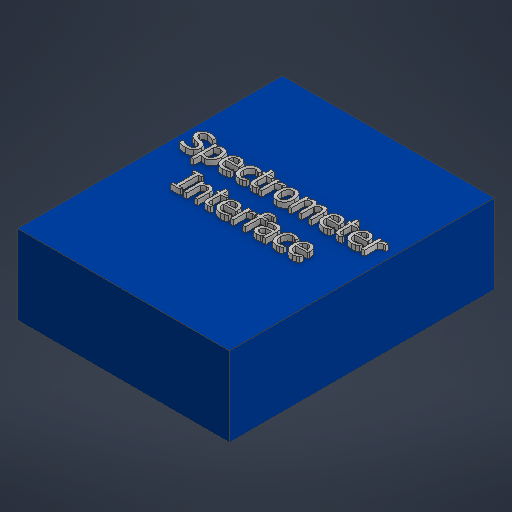
# Autodesk Inventor part: SpectrometerMeasurer
Saved by Autodesk Inventor 2025.1 (Build 291241000, 241)
## iProperties
Created: 2024-10-04
Part Number: SpectrometerMeasurer
Material: Generic
Document SubType Name: Modeling
Designer: jerem
Density: 1 g/cm^3
Appearance: Default
Author: jerem
Autodesk Inventor part; units mm, degrees
ref_plane "YZ Plane" through (0, 0, 0) normal (1, 0, 0) x (0, 1, 0)
ref_plane "XZ Plane" through (0, 0, 0) normal (0, 1, 0) x (-1, 0, 0)
ref_plane "XY Plane" through (0, 0, 0) normal (0, 0, 1) x (1, 0, 0)
sketch "Sketch1" plane through (0, 0, 0) normal (0, 1, 0) x (-1, 0, 0)
  line L0 (-40, -50) -> (40, -50)
  line L1 (40, -50) -> (40, 50)
  line L2 (40, 50) -> (-40, 50)
  line L3 (-40, 50) -> (-40, -50)
  line L4 (-40, -50) -> (40, 50) construction
  line L5 (40, -50) -> (-40, 50) construction
  point P0 (0, 0)
  dimension "d0" = 80
  dimension "d1" = 100
  constraints: 12 end point, 2 midpoint, 2 parallel, 1 horizontal, 1 perpendicular
  measures "d0" distance of L2.end L1.end
  measures "d1" distance of L1.end L0.end
extrude "Extrusion1" add sketch "Sketch1" along normal blind 30
sketch "Sketch2" plane through (0, 30, 0) normal (0, 1, 0) x (1, 0, 0)
  line L0 (-25.8871, 26.529) -> (26.7429, 26.529) construction
  line L1 (26.7429, 26.529) -> (26.7429, -19.6828) construction
  line L2 (26.7429, -19.6828) -> (-25.8871, -19.6828) construction
  line L3 (-25.8871, -19.6828) -> (-25.8871, 26.529) construction
  spline S0 degree 2 poles (-32.8043, 6.1864) (-33.7816, 6.1864) (-35.1527, 6.5948) (-35.7581, 6.8865) knots 0 0 0 1 2 2 2
  line L4 (-35.7581, 6.8865) -> (-35.7581, 8.389)
  line L5 (-35.7581, 8.389) -> (-35.6706, 8.389)
  spline S1 degree 2 poles (-35.6706, 8.389) (-35.0798, 7.8347) (-33.5847, 7.222) (-32.8918, 7.222) knots 0 0 0 1 2 2 2
  spline S2 degree 2 poles (-32.8918, 7.222) (-31.8999, 7.222) (-30.8861, 8.0462) (-30.8861, 8.7244) knots 0 0 0 1 2 2 2
  spline S3 degree 2 poles (-30.8861, 8.7244) (-30.8861, 9.2642) (-31.4185, 9.9351) (-31.9947, 10.1029) knots 0 0 0 1 2 2 2
  spline S4 degree 2 poles (-31.9947, 10.1029) (-32.4104, 10.2196) (-33.1033, 10.38) (-33.6211, 10.5113) knots 0 0 0 1 2 2 2
  spline S5 degree 2 poles (-33.6211, 10.5113) (-34.0879, 10.6353) (-34.8245, 11.0073) (-35.109, 11.3063) knots 0 0 0 1 2 2 2
  spline S6 degree 2 poles (-35.109, 11.3063) (-35.3861, 11.6053) (-35.6925, 12.4076) (-35.6925, 12.9327) knots 0 0 0 1 2 2 2
  spline S7 degree 2 poles (-35.6925, 12.9327) (-35.6925, 14.0267) (-33.9858, 15.5073) (-32.6657, 15.5073) knots 0 0 0 1 2 2 2
  spline S8 degree 2 poles (-32.6657, 15.5073) (-31.9072, 15.5073) (-30.5652, 15.2082) (-29.989, 14.9238) knots 0 0 0 1 2 2 2
  line L6 (-29.989, 14.9238) -> (-29.989, 13.4943)
  line L7 (-29.989, 13.4943) -> (-30.0766, 13.4943)
  spline S9 degree 2 poles (-30.0766, 13.4943) (-30.5069, 13.8881) (-31.8489, 14.4716) (-32.5855, 14.4716) knots 0 0 0 1 2 2 2
  spline S10 degree 2 poles (-32.5855, 14.4716) (-33.4169, 14.4716) (-34.4453, 13.6912) (-34.4453, 13.0567) knots 0 0 0 1 2 2 2
  spline S11 degree 2 poles (-34.4453, 13.0567) (-34.4453, 12.4878) (-33.8399, 11.8095) (-33.2711, 11.6564) knots 0 0 0 1 2 2 2
  spline S12 degree 2 poles (-33.2711, 11.6564) (-32.8918, 11.5543) (-31.7905, 11.2917) (-31.4258, 11.1823) knots 0 0 0 1 2 2 2
  spline S13 degree 2 poles (-31.4258, 11.1823) (-30.4996, 10.8979) (-29.639, 9.7528) (-29.639, 8.9141) knots 0 0 0 1 2 2 2
  spline S14 degree 2 poles (-29.639, 8.9141) (-29.639, 8.3817) (-30.0693, 7.3606) (-30.4558, 7.0032) knots 0 0 0 1 2 2 2
  spline S15 degree 2 poles (-30.4558, 7.0032) (-30.8861, 6.6094) (-31.9801, 6.1864) (-32.8043, 6.1864) knots 0 0 0 1 2 2 2
  spline S16 degree 2 poles (-22.8489, 9.906) (-22.8489, 8.2139) (-24.4607, 6.2155) (-25.6933, 6.2155) knots 0 0 0 1 2 2 2
  spline S17 degree 2 poles (-25.6933, 6.2155) (-26.1965, 6.2155) (-26.9696, 6.4489) (-27.3707, 6.6896) knots 0 0 0 1 2 2 2
  line L8 (-27.3707, 6.6896) -> (-27.3707, 3.8598)
  line L9 (-27.3707, 3.8598) -> (-28.5085, 3.8598)
  line L10 (-28.5085, 3.8598) -> (-28.5085, 13.1005)
  line L11 (-28.5085, 13.1005) -> (-27.3707, 13.1005)
  line L12 (-27.3707, 13.1005) -> (-27.3707, 12.393)
  spline S18 degree 2 poles (-27.3707, 12.393) (-26.9477, 12.7796) (-25.9121, 13.2901) (-25.3067, 13.2901) knots 0 0 0 1 2 2 2
  spline S19 degree 2 poles (-25.3067, 13.2901) (-24.1471, 13.2901) (-22.8489, 11.4522) (-22.8489, 9.906) knots 0 0 0 1 2 2 2
  spline S20 degree 2 poles (-24.0231, 9.7747) (-24.0231, 10.9343) (-24.7597, 12.2107) (-25.5839, 12.2107) knots 0 0 0 1 2 2 2
  spline S21 degree 2 poles (-25.5839, 12.2107) (-26.0652, 12.2107) (-26.9696, 11.7804) (-27.3707, 11.4449) knots 0 0 0 1 2 2 2
  line L13 (-27.3707, 11.4449) -> (-27.3707, 7.6086)
  spline S22 degree 2 poles (-27.3707, 7.6086) (-26.9258, 7.3971) (-26.2913, 7.2366) (-25.8829, 7.2366) knots 0 0 0 1 2 2 2
  spline S23 degree 2 poles (-25.8829, 7.2366) (-25.0004, 7.2366) (-24.0231, 8.5348) (-24.0231, 9.7747) knots 0 0 0 1 2 2 2
  spline S24 degree 2 poles (-18.7354, 6.1937) (-20.3545, 6.1937) (-22.1341, 8.0097) (-22.1341, 9.6872) knots 0 0 0 1 2 2 2
  spline S25 degree 2 poles (-22.1341, 9.6872) (-22.1341, 11.3355) (-20.4056, 13.2901) (-19.0125, 13.2901) knots 0 0 0 1 2 2 2
  spline S26 degree 2 poles (-19.0125, 13.2901) (-18.3853, 13.2901) (-17.4153, 12.9254) (-17.0579, 12.5389) knots 0 0 0 1 2 2 2
  spline S27 degree 2 poles (-17.0579, 12.5389) (-16.6933, 12.1523) (-16.3067, 11.0364) (-16.3067, 10.2269) knots 0 0 0 1 2 2 2
  line L14 (-16.3067, 10.2269) -> (-16.3067, 9.6069)
  line L15 (-16.3067, 9.6069) -> (-20.9818, 9.6069)
  spline S28 degree 2 poles (-20.9818, 9.6069) (-20.9818, 8.4327) (-19.8002, 7.1855) (-18.75, 7.1855) knots 0 0 0 1 2 2 2
  spline S29 degree 2 poles (-18.75, 7.1855) (-18.378, 7.1855) (-17.656, 7.3533) (-17.3643, 7.4846) knots 0 0 0 1 2 2 2
  spline S30 degree 2 poles (-17.3643, 7.4846) (-17.0579, 7.6304) (-16.6349, 7.8857) (-16.4963, 8.0024) knots 0 0 0 1 2 2 2
  line L16 (-16.4963, 8.0024) -> (-16.4307, 8.0024)
  line L17 (-16.4307, 8.0024) -> (-16.4307, 6.7625)
  spline S31 degree 2 poles (-16.4307, 6.7625) (-16.6276, 6.6823) (-17.2257, 6.4489) (-17.4591, 6.3833) knots 0 0 0 1 2 2 2
  spline S32 degree 2 poles (-17.4591, 6.3833) (-17.7873, 6.2885) (-18.327, 6.1937) (-18.7354, 6.1937) knots 0 0 0 1 2 2 2
  spline S33 degree 2 poles (-17.4153, 10.4749) (-17.4299, 10.9343) (-17.6195, 11.6053) (-17.8019, 11.8314) knots 0 0 0 1 2 2 2
  spline S34 degree 2 poles (-17.8019, 11.8314) (-17.9988, 12.0867) (-18.6187, 12.3565) (-19.0782, 12.3565) knots 0 0 0 1 2 2 2
  spline S35 degree 2 poles (-19.0782, 12.3565) (-19.5304, 12.3565) (-20.1649, 12.0867) (-20.4275, 11.8241) knots 0 0 0 1 2 2 2
  spline S36 degree 2 poles (-20.4275, 11.8241) (-20.6827, 11.5543) (-20.9453, 10.9052) (-20.9818, 10.4749) knots 0 0 0 1 2 2 2
  line L18 (-20.9818, 10.4749) -> (-17.4153, 10.4749)
  spline S37 degree 2 poles (-12.4704, 6.1937) (-13.1706, 6.1937) (-14.3302, 6.624) (-14.7459, 7.0616) knots 0 0 0 1 2 2 2
  spline S38 degree 2 poles (-14.7459, 7.0616) (-15.1617, 7.4919) (-15.6211, 8.8193) (-15.6211, 9.709) knots 0 0 0 1 2 2 2
  spline S39 degree 2 poles (-15.6211, 9.709) (-15.6211, 10.5988) (-15.1471, 11.8971) (-14.7459, 12.3347) knots 0 0 0 1 2 2 2
  spline S40 degree 2 poles (-14.7459, 12.3347) (-14.3448, 12.7796) (-13.156, 13.2536) (-12.4704, 13.2536) knots 0 0 0 1 2 2 2
  spline S41 degree 2 poles (-12.4704, 13.2536) (-11.9161, 13.2536) (-10.8805, 12.94) (-10.4793, 12.7358) knots 0 0 0 1 2 2 2
  line L19 (-10.4793, 12.7358) -> (-10.4793, 11.4595)
  line L20 (-10.4793, 11.4595) -> (-10.545, 11.4595)
  spline S42 degree 2 poles (-10.545, 11.4595) (-10.669, 11.5616) (-11.0482, 11.8241) (-11.3181, 11.9627) knots 0 0 0 1 2 2 2
  spline S43 degree 2 poles (-11.3181, 11.9627) (-11.5587, 12.0794) (-12.2006, 12.2617) (-12.4923, 12.2617) knots 0 0 0 1 2 2 2
  spline S44 degree 2 poles (-12.4923, 12.2617) (-13.3748, 12.2617) (-14.4469, 10.927) (-14.4469, 9.709) knots 0 0 0 1 2 2 2
  spline S45 degree 2 poles (-14.4469, 9.709) (-14.4469, 8.5202) (-13.4113, 7.1855) (-12.4923, 7.1855) knots 0 0 0 1 2 2 2
  spline S46 degree 2 poles (-12.4923, 7.1855) (-11.938, 7.1855) (-10.9315, 7.645) (-10.545, 8.0024) knots 0 0 0 1 2 2 2
  line L21 (-10.545, 8.0024) -> (-10.4793, 8.0024)
  line L22 (-10.4793, 8.0024) -> (-10.4793, 6.7261)
  spline S47 degree 2 poles (-10.4793, 6.7261) (-10.6471, 6.6458) (-11.1576, 6.4197) (-11.3618, 6.3687) knots 0 0 0 1 2 2 2
  spline S48 degree 2 poles (-11.3618, 6.3687) (-11.6536, 6.2812) (-12.113, 6.1937) (-12.4704, 6.1937) knots 0 0 0 1 2 2 2
  spline S49 degree 2 poles (-7.4015, 6.2155) (-8.3278, 6.2155) (-9.3707, 7.2731) (-9.3707, 8.4181) knots 0 0 0 1 2 2 2
  line L23 (-9.3707, 8.4181) -> (-9.3707, 12.1596)
  line L24 (-9.3707, 12.1596) -> (-10.1365, 12.1596)
  line L25 (-10.1365, 12.1596) -> (-10.1365, 13.1005)
  line L26 (-10.1365, 13.1005) -> (-9.3707, 13.1005)
  line L27 (-9.3707, 13.1005) -> (-9.3707, 15.0405)
  line L28 (-9.3707, 15.0405) -> (-8.233, 15.0405)
  line L29 (-8.233, 15.0405) -> (-8.233, 13.1005)
  line L30 (-8.233, 13.1005) -> (-6.1398, 13.1005)
  line L31 (-6.1398, 13.1005) -> (-6.1398, 12.1596)
  line L32 (-6.1398, 12.1596) -> (-8.233, 12.1596)
  line L33 (-8.233, 12.1596) -> (-8.233, 8.9432)
  spline S50 degree 2 poles (-8.233, 8.9432) (-8.233, 8.4327) (-8.1965, 7.8711) (-8.0725, 7.6304) knots 0 0 0 1 2 2 2
  spline S51 degree 2 poles (-8.0725, 7.6304) (-7.9704, 7.4189) (-7.5109, 7.2074) (-7.1171, 7.2074) knots 0 0 0 1 2 2 2
  spline S52 degree 2 poles (-7.1171, 7.2074) (-6.8399, 7.2074) (-6.3221, 7.3752) (-6.2054, 7.4262) knots 0 0 0 1 2 2 2
  line L34 (-6.2054, 7.4262) -> (-6.1398, 7.4262)
  line L35 (-6.1398, 7.4262) -> (-6.1398, 6.4052)
  spline S53 degree 2 poles (-6.1398, 6.4052) (-6.4607, 6.3176) (-7.1171, 6.2155) (-7.4015, 6.2155) knots 0 0 0 1 2 2 2
  line L36 (-1.72, 11.8825) -> (-1.7784, 11.8825)
  spline S54 degree 2 poles (-1.7784, 11.8825) (-1.9096, 11.9189) (-2.1941, 11.9335) (-2.391, 11.9335) knots 0 0 0 1 2 2 2
  spline S55 degree 2 poles (-2.391, 11.9335) (-2.8505, 11.9335) (-3.7549, 11.5324) (-4.1633, 11.1385) knots 0 0 0 1 2 2 2
  line L37 (-4.1633, 11.1385) -> (-4.1633, 6.3468)
  line L38 (-4.1633, 6.3468) -> (-5.301, 6.3468)
  line L39 (-5.301, 6.3468) -> (-5.301, 13.1005)
  line L40 (-5.301, 13.1005) -> (-4.1633, 13.1005)
  line L41 (-4.1633, 13.1005) -> (-4.1633, 12.094)
  spline S56 degree 2 poles (-4.1633, 12.094) (-3.5433, 12.6483) (-2.6171, 13.1005) (-2.1795, 13.1005) knots 0 0 0 1 2 2 2
  spline S57 degree 2 poles (-2.1795, 13.1005) (-2.0044, 13.1005) (-1.8294, 13.0859) (-1.72, 13.064) knots 0 0 0 1 2 2 2
  line L42 (-1.72, 13.064) -> (-1.72, 11.8825)
  spline S58 degree 2 poles (4.7127, 9.7236) (4.7127, 8.017) (3.0717, 6.1572) (1.7006, 6.1572) knots 0 0 0 1 2 2 2
  spline S59 degree 2 poles (1.7006, 6.1572) (0.293, 6.1572) (-1.3189, 8.0753) (-1.3189, 9.7236) knots 0 0 0 1 2 2 2
  spline S60 degree 2 poles (-1.3189, 9.7236) (-1.3189, 11.4157) (0.344, 13.2901) (1.7006, 13.2901) knots 0 0 0 1 2 2 2
  spline S61 degree 2 poles (1.7006, 13.2901) (3.0717, 13.2901) (4.7127, 11.423) (4.7127, 9.7236) knots 0 0 0 1 2 2 2
  spline S62 degree 2 poles (3.5385, 9.7236) (3.5385, 11.0364) (2.5831, 12.3128) (1.7006, 12.3128) knots 0 0 0 1 2 2 2
  spline S63 degree 2 poles (1.7006, 12.3128) (0.8181, 12.3128) (-0.1446, 11.0364) (-0.1446, 9.7236) knots 0 0 0 1 2 2 2
  spline S64 degree 2 poles (-0.1446, 9.7236) (-0.1446, 8.4473) (0.8181, 7.1345) (1.7006, 7.1345) knots 0 0 0 1 2 2 2
  spline S65 degree 2 poles (1.7006, 7.1345) (2.5758, 7.1345) (3.5385, 8.4254) (3.5385, 9.7236) knots 0 0 0 1 2 2 2
  line L43 (13.5377, 6.3468) -> (13.5377, 10.256)
  spline S66 degree 2 poles (13.5377, 10.256) (13.5377, 10.7228) (13.4648, 11.5178) (13.3481, 11.7366) knots 0 0 0 1 2 2 2
  spline S67 degree 2 poles (13.3481, 11.7366) (13.2314, 11.9773) (12.7865, 12.2107) (12.3999, 12.2107) knots 0 0 0 1 2 2 2
  spline S68 degree 2 poles (12.3999, 12.2107) (12.0498, 12.2107) (11.2476, 11.7804) (10.8246, 11.3719) knots 0 0 0 1 2 2 2
  spline S69 degree 2 poles (10.8246, 11.3719) (10.8319, 11.2698) (10.8464, 10.9854) (10.8464, 10.7958) knots 0 0 0 1 2 2 2
  line L44 (10.8464, 10.7958) -> (10.8464, 6.3468)
  line L45 (10.8464, 6.3468) -> (9.7087, 6.3468)
  line L46 (9.7087, 6.3468) -> (9.7087, 10.256)
  spline S70 degree 2 poles (9.7087, 10.256) (9.7087, 10.7228) (9.6357, 11.5178) (9.5191, 11.7366) knots 0 0 0 1 2 2 2
  spline S71 degree 2 poles (9.5191, 11.7366) (9.4024, 11.9773) (8.9575, 12.2107) (8.5709, 12.2107) knots 0 0 0 1 2 2 2
  spline S72 degree 2 poles (8.5709, 12.2107) (8.2063, 12.2107) (7.3967, 11.7512) (7.0174, 11.3938) knots 0 0 0 1 2 2 2
  line L47 (7.0174, 11.3938) -> (7.0174, 6.3468)
  line L48 (7.0174, 6.3468) -> (5.8797, 6.3468)
  line L49 (5.8797, 6.3468) -> (5.8797, 13.1005)
  line L50 (5.8797, 13.1005) -> (7.0174, 13.1005)
  line L51 (7.0174, 13.1005) -> (7.0174, 12.3565)
  spline S73 degree 2 poles (7.0174, 12.3565) (7.4623, 12.8014) (8.3375, 13.2901) (8.8627, 13.2901) knots 0 0 0 1 2 2 2
  spline S74 degree 2 poles (8.8627, 13.2901) (9.4607, 13.2901) (10.387, 12.7431) (10.6276, 12.1231) knots 0 0 0 1 2 2 2
  spline S75 degree 2 poles (10.6276, 12.1231) (11.1455, 12.6993) (12.1228, 13.2901) (12.6917, 13.2901) knots 0 0 0 1 2 2 2
  spline S76 degree 2 poles (12.6917, 13.2901) (13.1293, 13.2901) (13.844, 13.0202) (14.1066, 12.7139) knots 0 0 0 1 2 2 2
  spline S77 degree 2 poles (14.1066, 12.7139) (14.3764, 12.4076) (14.6755, 11.4886) (14.6755, 10.7958) knots 0 0 0 1 2 2 2
  line L52 (14.6755, 10.7958) -> (14.6755, 6.3468)
  line L53 (14.6755, 6.3468) -> (13.5377, 6.3468)
  spline S78 degree 2 poles (19.2046, 6.1937) (17.5855, 6.1937) (15.8059, 8.0097) (15.8059, 9.6872) knots 0 0 0 1 2 2 2
  spline S79 degree 2 poles (15.8059, 9.6872) (15.8059, 11.3355) (17.5345, 13.2901) (18.9275, 13.2901) knots 0 0 0 1 2 2 2
  spline S80 degree 2 poles (18.9275, 13.2901) (19.5547, 13.2901) (20.5247, 12.9254) (20.8821, 12.5389) knots 0 0 0 1 2 2 2
  spline S81 degree 2 poles (20.8821, 12.5389) (21.2468, 12.1523) (21.6333, 11.0364) (21.6333, 10.2269) knots 0 0 0 1 2 2 2
  line L54 (21.6333, 10.2269) -> (21.6333, 9.6069)
  line L55 (21.6333, 9.6069) -> (16.9583, 9.6069)
  spline S82 degree 2 poles (16.9583, 9.6069) (16.9583, 8.4327) (18.1398, 7.1855) (19.19, 7.1855) knots 0 0 0 1 2 2 2
  spline S83 degree 2 poles (19.19, 7.1855) (19.562, 7.1855) (20.284, 7.3533) (20.5758, 7.4846) knots 0 0 0 1 2 2 2
  spline S84 degree 2 poles (20.5758, 7.4846) (20.8821, 7.6304) (21.3051, 7.8857) (21.4437, 8.0024) knots 0 0 0 1 2 2 2
  line L56 (21.4437, 8.0024) -> (21.5093, 8.0024)
  line L57 (21.5093, 8.0024) -> (21.5093, 6.7625)
  spline S85 degree 2 poles (21.5093, 6.7625) (21.3124, 6.6823) (20.7144, 6.4489) (20.481, 6.3833) knots 0 0 0 1 2 2 2
  spline S86 degree 2 poles (20.481, 6.3833) (20.1528, 6.2885) (19.6131, 6.1937) (19.2046, 6.1937) knots 0 0 0 1 2 2 2
  spline S87 degree 2 poles (20.5247, 10.4749) (20.5101, 10.9343) (20.3205, 11.6053) (20.1382, 11.8314) knots 0 0 0 1 2 2 2
  spline S88 degree 2 poles (20.1382, 11.8314) (19.9413, 12.0867) (19.3213, 12.3565) (18.8618, 12.3565) knots 0 0 0 1 2 2 2
  spline S89 degree 2 poles (18.8618, 12.3565) (18.4097, 12.3565) (17.7751, 12.0867) (17.5126, 11.8241) knots 0 0 0 1 2 2 2
  spline S90 degree 2 poles (17.5126, 11.8241) (17.2573, 11.5543) (16.9947, 10.9052) (16.9583, 10.4749) knots 0 0 0 1 2 2 2
  line L58 (16.9583, 10.4749) -> (20.5247, 10.4749)
  spline S91 degree 2 poles (24.8278, 6.2155) (23.9015, 6.2155) (22.8586, 7.2731) (22.8586, 8.4181) knots 0 0 0 1 2 2 2
  line L59 (22.8586, 8.4181) -> (22.8586, 12.1596)
  line L60 (22.8586, 12.1596) -> (22.0928, 12.1596)
  line L61 (22.0928, 12.1596) -> (22.0928, 13.1005)
  line L62 (22.0928, 13.1005) -> (22.8586, 13.1005)
  line L63 (22.8586, 13.1005) -> (22.8586, 15.0405)
  line L64 (22.8586, 15.0405) -> (23.9964, 15.0405)
  line L65 (23.9964, 15.0405) -> (23.9964, 13.1005)
  line L66 (23.9964, 13.1005) -> (26.0896, 13.1005)
  line L67 (26.0896, 13.1005) -> (26.0896, 12.1596)
  line L68 (26.0896, 12.1596) -> (23.9964, 12.1596)
  line L69 (23.9964, 12.1596) -> (23.9964, 8.9432)
  spline S92 degree 2 poles (23.9964, 8.9432) (23.9964, 8.4327) (24.0328, 7.8711) (24.1568, 7.6304) knots 0 0 0 1 2 2 2
  spline S93 degree 2 poles (24.1568, 7.6304) (24.2589, 7.4189) (24.7184, 7.2074) (25.1122, 7.2074) knots 0 0 0 1 2 2 2
  spline S94 degree 2 poles (25.1122, 7.2074) (25.3894, 7.2074) (25.9072, 7.3752) (26.0239, 7.4262) knots 0 0 0 1 2 2 2
  line L70 (26.0239, 7.4262) -> (26.0896, 7.4262)
  line L71 (26.0896, 7.4262) -> (26.0896, 6.4052)
  spline S95 degree 2 poles (26.0896, 6.4052) (25.7686, 6.3176) (25.1122, 6.2155) (24.8278, 6.2155) knots 0 0 0 1 2 2 2
  spline S96 degree 2 poles (29.8602, 6.1937) (28.2411, 6.1937) (26.4615, 8.0097) (26.4615, 9.6872) knots 0 0 0 1 2 2 2
  spline S97 degree 2 poles (26.4615, 9.6872) (26.4615, 11.3355) (28.19, 13.2901) (29.5831, 13.2901) knots 0 0 0 1 2 2 2
  spline S98 degree 2 poles (29.5831, 13.2901) (30.2103, 13.2901) (31.1803, 12.9254) (31.5377, 12.5389) knots 0 0 0 1 2 2 2
  spline S99 degree 2 poles (31.5377, 12.5389) (31.9024, 12.1523) (32.2889, 11.0364) (32.2889, 10.2269) knots 0 0 0 1 2 2 2
  line L72 (32.2889, 10.2269) -> (32.2889, 9.6069)
  line L73 (32.2889, 9.6069) -> (27.6139, 9.6069)
  spline S100 degree 2 poles (27.6139, 9.6069) (27.6139, 8.4327) (28.7954, 7.1855) (29.8456, 7.1855) knots 0 0 0 1 2 2 2
  spline S101 degree 2 poles (29.8456, 7.1855) (30.2176, 7.1855) (30.9396, 7.3533) (31.2314, 7.4846) knots 0 0 0 1 2 2 2
  spline S102 degree 2 poles (31.2314, 7.4846) (31.5377, 7.6304) (31.9607, 7.8857) (32.0993, 8.0024) knots 0 0 0 1 2 2 2
  line L74 (32.0993, 8.0024) -> (32.1649, 8.0024)
  line L75 (32.1649, 8.0024) -> (32.1649, 6.7625)
  spline S103 degree 2 poles (32.1649, 6.7625) (31.968, 6.6823) (31.3699, 6.4489) (31.1366, 6.3833) knots 0 0 0 1 2 2 2
  spline S104 degree 2 poles (31.1366, 6.3833) (30.8084, 6.2885) (30.2686, 6.1937) (29.8602, 6.1937) knots 0 0 0 1 2 2 2
  spline S105 degree 2 poles (31.1803, 10.4749) (31.1657, 10.9343) (30.9761, 11.6053) (30.7938, 11.8314) knots 0 0 0 1 2 2 2
  spline S106 degree 2 poles (30.7938, 11.8314) (30.5968, 12.0867) (29.9769, 12.3565) (29.5174, 12.3565) knots 0 0 0 1 2 2 2
  spline S107 degree 2 poles (29.5174, 12.3565) (29.0652, 12.3565) (28.4307, 12.0867) (28.1682, 11.8241) knots 0 0 0 1 2 2 2
  spline S108 degree 2 poles (28.1682, 11.8241) (27.9129, 11.5543) (27.6503, 10.9052) (27.6139, 10.4749) knots 0 0 0 1 2 2 2
  line L76 (27.6139, 10.4749) -> (31.1803, 10.4749)
  line L77 (37.0223, 11.8825) -> (36.9639, 11.8825)
  spline S109 degree 2 poles (36.9639, 11.8825) (36.8327, 11.9189) (36.5482, 11.9335) (36.3513, 11.9335) knots 0 0 0 1 2 2 2
  spline S110 degree 2 poles (36.3513, 11.9335) (35.8918, 11.9335) (34.9874, 11.5324) (34.579, 11.1385) knots 0 0 0 1 2 2 2
  line L78 (34.579, 11.1385) -> (34.579, 6.3468)
  line L79 (34.579, 6.3468) -> (33.4413, 6.3468)
  line L80 (33.4413, 6.3468) -> (33.4413, 13.1005)
  line L81 (33.4413, 13.1005) -> (34.579, 13.1005)
  line L82 (34.579, 13.1005) -> (34.579, 12.094)
  spline S111 degree 2 poles (34.579, 12.094) (35.199, 12.6483) (36.1252, 13.1005) (36.5628, 13.1005) knots 0 0 0 1 2 2 2
  spline S112 degree 2 poles (36.5628, 13.1005) (36.7379, 13.1005) (36.9129, 13.0859) (37.0223, 13.064) knots 0 0 0 1 2 2 2
  line L83 (37.0223, 13.064) -> (37.0223, 11.8825)
  line L84 (-20.1722, -8.4715) -> (-23.6584, -8.4715)
  line L85 (-23.6584, -8.4715) -> (-23.6584, -7.5525)
  line L86 (-23.6584, -7.5525) -> (-22.5134, -7.5525)
  line L87 (-22.5134, -7.5525) -> (-22.5134, -0.3904)
  line L88 (-22.5134, -0.3904) -> (-23.6584, -0.3904)
  line L89 (-23.6584, -0.3904) -> (-23.6584, 0.5285)
  line L90 (-23.6584, 0.5285) -> (-20.1722, 0.5285)
  line L91 (-20.1722, 0.5285) -> (-20.1722, -0.3904)
  line L92 (-20.1722, -0.3904) -> (-21.3172, -0.3904)
  line L93 (-21.3172, -0.3904) -> (-21.3172, -7.5525)
  line L94 (-21.3172, -7.5525) -> (-20.1722, -7.5525)
  line L95 (-20.1722, -7.5525) -> (-20.1722, -8.4715)
  line L96 (-13.4769, -8.4715) -> (-14.6147, -8.4715)
  line L97 (-14.6147, -8.4715) -> (-14.6147, -4.6206)
  spline S113 degree 2 poles (-14.6147, -4.6206) (-14.6147, -4.1538) (-14.7022, -3.3515) (-14.8335, -3.1108) knots 0 0 0 1 2 2 2
  spline S114 degree 2 poles (-14.8335, -3.1108) (-14.972, -2.8556) (-15.468, -2.6076) (-15.891, -2.6076) knots 0 0 0 1 2 2 2
  spline S115 degree 2 poles (-15.891, -2.6076) (-16.314, -2.6076) (-17.2111, -3.0598) (-17.6414, -3.4244) knots 0 0 0 1 2 2 2
  line L98 (-17.6414, -3.4244) -> (-17.6414, -8.4715)
  line L99 (-17.6414, -8.4715) -> (-18.7792, -8.4715)
  line L100 (-18.7792, -8.4715) -> (-18.7792, -1.7178)
  line L101 (-18.7792, -1.7178) -> (-17.6414, -1.7178)
  line L102 (-17.6414, -1.7178) -> (-17.6414, -2.469)
  spline S116 degree 2 poles (-17.6414, -2.469) (-17.1309, -2.0095) (-16.1463, -1.5282) (-15.592, -1.5282) knots 0 0 0 1 2 2 2
  spline S117 degree 2 poles (-15.592, -1.5282) (-14.6001, -1.5282) (-13.4769, -2.841) (-13.4769, -4.0881) knots 0 0 0 1 2 2 2
  line L103 (-13.4769, -4.0881) -> (-13.4769, -8.4715)
  spline S118 degree 2 poles (-9.8375, -8.6027) (-10.7638, -8.6027) (-11.8067, -7.5452) (-11.8067, -6.4001) knots 0 0 0 1 2 2 2
  line L104 (-11.8067, -6.4001) -> (-11.8067, -2.6586)
  line L105 (-11.8067, -2.6586) -> (-12.5725, -2.6586)
  line L106 (-12.5725, -2.6586) -> (-12.5725, -1.7178)
  line L107 (-12.5725, -1.7178) -> (-11.8067, -1.7178)
  line L108 (-11.8067, -1.7178) -> (-11.8067, 0.2222)
  line L109 (-11.8067, 0.2222) -> (-10.669, 0.2222)
  line L110 (-10.669, 0.2222) -> (-10.669, -1.7178)
  line L111 (-10.669, -1.7178) -> (-8.5758, -1.7178)
  line L112 (-8.5758, -1.7178) -> (-8.5758, -2.6586)
  line L113 (-8.5758, -2.6586) -> (-10.669, -2.6586)
  line L114 (-10.669, -2.6586) -> (-10.669, -5.875)
  spline S119 degree 2 poles (-10.669, -5.875) (-10.669, -6.3856) (-10.6325, -6.9471) (-10.5085, -7.1878) knots 0 0 0 1 2 2 2
  spline S120 degree 2 poles (-10.5085, -7.1878) (-10.4064, -7.3993) (-9.9469, -7.6108) (-9.5531, -7.6108) knots 0 0 0 1 2 2 2
  spline S121 degree 2 poles (-9.5531, -7.6108) (-9.2759, -7.6108) (-8.7581, -7.4431) (-8.6414, -7.392) knots 0 0 0 1 2 2 2
  line L115 (-8.6414, -7.392) -> (-8.5758, -7.392)
  line L116 (-8.5758, -7.392) -> (-8.5758, -8.4131)
  spline S122 degree 2 poles (-8.5758, -8.4131) (-8.8967, -8.5006) (-9.5531, -8.6027) (-9.8375, -8.6027) knots 0 0 0 1 2 2 2
  spline S123 degree 2 poles (-4.8051, -8.6246) (-6.4242, -8.6246) (-8.2038, -6.8086) (-8.2038, -5.1311) knots 0 0 0 1 2 2 2
  spline S124 degree 2 poles (-8.2038, -5.1311) (-8.2038, -3.4828) (-6.4753, -1.5282) (-5.0822, -1.5282) knots 0 0 0 1 2 2 2
  spline S125 degree 2 poles (-5.0822, -1.5282) (-4.455, -1.5282) (-3.485, -1.8928) (-3.1276, -2.2794) knots 0 0 0 1 2 2 2
  spline S126 degree 2 poles (-3.1276, -2.2794) (-2.763, -2.6659) (-2.3764, -3.7818) (-2.3764, -4.5914) knots 0 0 0 1 2 2 2
  line L117 (-2.3764, -4.5914) -> (-2.3764, -5.2113)
  line L118 (-2.3764, -5.2113) -> (-7.0514, -5.2113)
  spline S127 degree 2 poles (-7.0514, -5.2113) (-7.0514, -6.3856) (-5.8699, -7.6327) (-4.8197, -7.6327) knots 0 0 0 1 2 2 2
  spline S128 degree 2 poles (-4.8197, -7.6327) (-4.4477, -7.6327) (-3.7257, -7.465) (-3.4339, -7.3337) knots 0 0 0 1 2 2 2
  spline S129 degree 2 poles (-3.4339, -7.3337) (-3.1276, -7.1878) (-2.7046, -6.9326) (-2.566, -6.8159) knots 0 0 0 1 2 2 2
  line L119 (-2.566, -6.8159) -> (-2.5004, -6.8159)
  line L120 (-2.5004, -6.8159) -> (-2.5004, -8.0557)
  spline S130 degree 2 poles (-2.5004, -8.0557) (-2.6973, -8.136) (-3.2954, -8.3693) (-3.5288, -8.435) knots 0 0 0 1 2 2 2
  spline S131 degree 2 poles (-3.5288, -8.435) (-3.857, -8.5298) (-4.3967, -8.6246) (-4.8051, -8.6246) knots 0 0 0 1 2 2 2
  spline S132 degree 2 poles (-3.485, -4.3434) (-3.4996, -3.8839) (-3.6892, -3.2129) (-3.8715, -2.9868) knots 0 0 0 1 2 2 2
  spline S133 degree 2 poles (-3.8715, -2.9868) (-4.0685, -2.7316) (-4.6884, -2.4617) (-5.1479, -2.4617) knots 0 0 0 1 2 2 2
  spline S134 degree 2 poles (-5.1479, -2.4617) (-5.6001, -2.4617) (-6.2346, -2.7316) (-6.4972, -2.9941) knots 0 0 0 1 2 2 2
  spline S135 degree 2 poles (-6.4972, -2.9941) (-6.7524, -3.264) (-7.015, -3.9131) (-7.0514, -4.3434) knots 0 0 0 1 2 2 2
  line L121 (-7.0514, -4.3434) -> (-3.485, -4.3434)
  line L122 (2.357, -2.9358) -> (2.2986, -2.9358)
  spline S136 degree 2 poles (2.2986, -2.9358) (2.1674, -2.8993) (1.8829, -2.8847) (1.686, -2.8847) knots 0 0 0 1 2 2 2
  spline S137 degree 2 poles (1.686, -2.8847) (1.2265, -2.8847) (0.3221, -3.2859) (-0.0863, -3.6797) knots 0 0 0 1 2 2 2
  line L123 (-0.0863, -3.6797) -> (-0.0863, -8.4715)
  line L124 (-0.0863, -8.4715) -> (-1.2241, -8.4715)
  line L125 (-1.2241, -8.4715) -> (-1.2241, -1.7178)
  line L126 (-1.2241, -1.7178) -> (-0.0863, -1.7178)
  line L127 (-0.0863, -1.7178) -> (-0.0863, -2.7243)
  spline S138 degree 2 poles (-0.0863, -2.7243) (0.5336, -2.17) (1.4599, -1.7178) (1.8975, -1.7178) knots 0 0 0 1 2 2 2
  spline S139 degree 2 poles (1.8975, -1.7178) (2.0725, -1.7178) (2.2476, -1.7324) (2.357, -1.7543) knots 0 0 0 1 2 2 2
  line L128 (2.357, -1.7543) -> (2.357, -2.9358)
  line L129 (6.7913, -0.1643) -> (6.733, -0.1643)
  spline S140 degree 2 poles (6.733, -0.1643) (6.5798, -0.106) (6.011, -0.0039) (5.7849, -0.0039) knots 0 0 0 1 2 2 2
  spline S141 degree 2 poles (5.7849, -0.0039) (5.0701, -0.0039) (4.4575, -0.6457) (4.4575, -1.4917) knots 0 0 0 1 2 2 2
  line L130 (4.4575, -1.4917) -> (4.4575, -1.7178)
  line L131 (4.4575, -1.7178) -> (6.3392, -1.7178)
  line L132 (6.3392, -1.7178) -> (6.3392, -2.6586)
  line L133 (6.3392, -2.6586) -> (4.4939, -2.6586)
  line L134 (4.4939, -2.6586) -> (4.4939, -8.4715)
  line L135 (4.4939, -8.4715) -> (3.3562, -8.4715)
  line L136 (3.3562, -8.4715) -> (3.3562, -2.6586)
  line L137 (3.3562, -2.6586) -> (2.5904, -2.6586)
  line L138 (2.5904, -2.6586) -> (2.5904, -1.7178)
  line L139 (2.5904, -1.7178) -> (3.3562, -1.7178)
  line L140 (3.3562, -1.7178) -> (3.3562, -1.4917)
  spline S142 degree 2 poles (3.3562, -1.4917) (3.3562, -0.281) (4.5304, 0.988) (5.6244, 0.988) knots 0 0 0 1 2 2 2
  spline S143 degree 2 poles (5.6244, 0.988) (5.938, 0.988) (6.5434, 0.9224) (6.7913, 0.8786) knots 0 0 0 1 2 2 2
  line L141 (6.7913, 0.8786) -> (6.7913, -0.1643)
  spline S144 degree 2 poles (10.9413, -7.7567) (10.8027, -7.8588) (10.3359, -8.2235) (10.1171, -8.3329) knots 0 0 0 1 2 2 2
  spline S145 degree 2 poles (10.1171, -8.3329) (9.8181, -8.4933) (9.2565, -8.6611) (8.746, -8.6611) knots 0 0 0 1 2 2 2
  spline S146 degree 2 poles (8.746, -8.6611) (8.3302, -8.6611) (7.579, -8.3475) (7.2946, -8.063) knots 0 0 0 1 2 2 2
  spline S147 degree 2 poles (7.2946, -8.063) (7.0247, -7.7859) (6.6965, -6.969) (6.6965, -6.5168) knots 0 0 0 1 2 2 2
  spline S148 degree 2 poles (6.6965, -6.5168) (6.6965, -5.8167) (7.2873, -4.8248) (7.9291, -4.5403) knots 0 0 0 1 2 2 2
  spline S149 degree 2 poles (7.9291, -4.5403) (8.498, -4.2778) (10.0442, -4.0809) (10.9413, -4.0298) knots 0 0 0 1 2 2 2
  line L142 (10.9413, -4.0298) -> (10.9413, -3.811)
  spline S150 degree 2 poles (10.9413, -3.811) (10.9413, -3.4172) (10.7006, -2.9285) (10.4818, -2.7899) knots 0 0 0 1 2 2 2
  spline S151 degree 2 poles (10.4818, -2.7899) (10.263, -2.6514) (9.6357, -2.5638) (9.3003, -2.5638) knots 0 0 0 1 2 2 2
  spline S152 degree 2 poles (9.3003, -2.5638) (8.9064, -2.5638) (7.8416, -2.7972) (7.3092, -3.0233) knots 0 0 0 1 2 2 2
  line L143 (7.3092, -3.0233) -> (7.2435, -3.0233)
  line L144 (7.2435, -3.0233) -> (7.2435, -1.8637)
  spline S153 degree 2 poles (7.2435, -1.8637) (7.5571, -1.7762) (8.7314, -1.5574) (9.3075, -1.5574) knots 0 0 0 1 2 2 2
  spline S154 degree 2 poles (9.3075, -1.5574) (10.0077, -1.5574) (10.9631, -1.7762) (11.3424, -2.0606) knots 0 0 0 1 2 2 2
  spline S155 degree 2 poles (11.3424, -2.0606) (11.7144, -2.3377) (12.079, -3.2202) (12.079, -3.8548) knots 0 0 0 1 2 2 2
  line L145 (12.079, -3.8548) -> (12.079, -8.4715)
  line L146 (12.079, -8.4715) -> (10.9413, -8.4715)
  line L147 (10.9413, -8.4715) -> (10.9413, -7.7567)
  line L148 (10.9413, -6.8086) -> (10.9413, -4.9342)
  spline S156 degree 2 poles (10.9413, -4.9342) (10.5328, -4.9706) (9.3003, -5.0946) (8.9137, -5.2113) knots 0 0 0 1 2 2 2
  spline S157 degree 2 poles (8.9137, -5.2113) (8.4615, -5.3499) (7.8708, -5.9261) (7.8708, -6.4366) knots 0 0 0 1 2 2 2
  spline S158 degree 2 poles (7.8708, -6.4366) (7.8708, -7.0201) (8.5272, -7.6108) (9.1544, -7.6108) knots 0 0 0 1 2 2 2
  spline S159 degree 2 poles (9.1544, -7.6108) (9.6868, -7.6108) (10.562, -7.1514) (10.9413, -6.8086) knots 0 0 0 1 2 2 2
  spline S160 degree 2 poles (16.3602, -8.6246) (15.6601, -8.6246) (14.5004, -8.1943) (14.0847, -7.7567) knots 0 0 0 1 2 2 2
  spline S161 degree 2 poles (14.0847, -7.7567) (13.669, -7.3264) (13.2095, -5.999) (13.2095, -5.1092) knots 0 0 0 1 2 2 2
  spline S162 degree 2 poles (13.2095, -5.1092) (13.2095, -4.2194) (13.6836, -2.9212) (14.0847, -2.4836) knots 0 0 0 1 2 2 2
  spline S163 degree 2 poles (14.0847, -2.4836) (14.4858, -2.0387) (15.6746, -1.5646) (16.3602, -1.5646) knots 0 0 0 1 2 2 2
  spline S164 degree 2 poles (16.3602, -1.5646) (16.9145, -1.5646) (17.9502, -1.8783) (18.3513, -2.0825) knots 0 0 0 1 2 2 2
  line L149 (18.3513, -2.0825) -> (18.3513, -3.3588)
  line L150 (18.3513, -3.3588) -> (18.2857, -3.3588)
  spline S165 degree 2 poles (18.2857, -3.3588) (18.1617, -3.2567) (17.7824, -2.9941) (17.5126, -2.8556) knots 0 0 0 1 2 2 2
  spline S166 degree 2 poles (17.5126, -2.8556) (17.2719, -2.7389) (16.6301, -2.5565) (16.3383, -2.5565) knots 0 0 0 1 2 2 2
  spline S167 degree 2 poles (16.3383, -2.5565) (15.4558, -2.5565) (14.3837, -3.8912) (14.3837, -5.1092) knots 0 0 0 1 2 2 2
  spline S168 degree 2 poles (14.3837, -5.1092) (14.3837, -6.298) (15.4194, -7.6327) (16.3383, -7.6327) knots 0 0 0 1 2 2 2
  spline S169 degree 2 poles (16.3383, -7.6327) (16.8926, -7.6327) (17.8991, -7.1732) (18.2857, -6.8159) knots 0 0 0 1 2 2 2
  line L151 (18.2857, -6.8159) -> (18.3513, -6.8159)
  line L152 (18.3513, -6.8159) -> (18.3513, -8.0922)
  spline S170 degree 2 poles (18.3513, -8.0922) (18.1836, -8.1724) (17.673, -8.3985) (17.4688, -8.4496) knots 0 0 0 1 2 2 2
  spline S171 degree 2 poles (17.4688, -8.4496) (17.1771, -8.5371) (16.7176, -8.6246) (16.3602, -8.6246) knots 0 0 0 1 2 2 2
  spline S172 degree 2 poles (22.3189, -8.6246) (20.6998, -8.6246) (18.9202, -6.8086) (18.9202, -5.1311) knots 0 0 0 1 2 2 2
  spline S173 degree 2 poles (18.9202, -5.1311) (18.9202, -3.4828) (20.6487, -1.5282) (22.0417, -1.5282) knots 0 0 0 1 2 2 2
  spline S174 degree 2 poles (22.0417, -1.5282) (22.669, -1.5282) (23.639, -1.8928) (23.9964, -2.2794) knots 0 0 0 1 2 2 2
  spline S175 degree 2 poles (23.9964, -2.2794) (24.361, -2.6659) (24.7476, -3.7818) (24.7476, -4.5914) knots 0 0 0 1 2 2 2
  line L153 (24.7476, -4.5914) -> (24.7476, -5.2113)
  line L154 (24.7476, -5.2113) -> (20.0725, -5.2113)
  spline S176 degree 2 poles (20.0725, -5.2113) (20.0725, -6.3856) (21.2541, -7.6327) (22.3043, -7.6327) knots 0 0 0 1 2 2 2
  spline S177 degree 2 poles (22.3043, -7.6327) (22.6763, -7.6327) (23.3983, -7.465) (23.69, -7.3337) knots 0 0 0 1 2 2 2
  spline S178 degree 2 poles (23.69, -7.3337) (23.9964, -7.1878) (24.4194, -6.9326) (24.558, -6.8159) knots 0 0 0 1 2 2 2
  line L155 (24.558, -6.8159) -> (24.6236, -6.8159)
  line L156 (24.6236, -6.8159) -> (24.6236, -8.0557)
  spline S179 degree 2 poles (24.6236, -8.0557) (24.4267, -8.136) (23.8286, -8.3693) (23.5952, -8.435) knots 0 0 0 1 2 2 2
  spline S180 degree 2 poles (23.5952, -8.435) (23.267, -8.5298) (22.7273, -8.6246) (22.3189, -8.6246) knots 0 0 0 1 2 2 2
  spline S181 degree 2 poles (23.639, -4.3434) (23.6244, -3.8839) (23.4348, -3.2129) (23.2524, -2.9868) knots 0 0 0 1 2 2 2
  spline S182 degree 2 poles (23.2524, -2.9868) (23.0555, -2.7316) (22.4356, -2.4617) (21.9761, -2.4617) knots 0 0 0 1 2 2 2
  spline S183 degree 2 poles (21.9761, -2.4617) (21.5239, -2.4617) (20.8894, -2.7316) (20.6268, -2.9941) knots 0 0 0 1 2 2 2
  spline S184 degree 2 poles (20.6268, -2.9941) (20.3716, -3.264) (20.109, -3.9131) (20.0725, -4.3434) knots 0 0 0 1 2 2 2
  line L157 (20.0725, -4.3434) -> (23.639, -4.3434)
  point P0 (0, 0)
  constraints: 2 other
extrude "Extrusion2" add sketch "Sketch2" along normal blind 2
body "Solid1"
